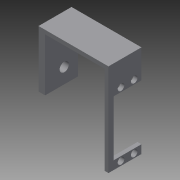
# Autodesk Inventor part: new_shoulder_2_modif
Saved by Autodesk Inventor 2014 SP1 (Build 180222100, 222)
## iProperties
Created: 2014-12-06
Part Number: new_shoulder_2_modif
Material: Générique
Document SubType Name: Modeling
Designer: astralien3000
Density: 1 g/cm^3
Appearance: Par défaut
d0: 45,000 mm
d1: 5,000 mm
d2: 3,000 mm
d3: 3,000 mm
d4: 40,000 mm
d5: 20,000 mm
d6: 22,500 mm
d7: 70,000 mm
d8: 25,000 mm
d9: 0,00 deg
d10: 21,000 mm
d11: 6,400 mm
d12: 6,400 mm
d13: 42,000 mm
d14: 5,000 mm
d15: 5,000 mm
d16: 5,000 mm
d17: 3,200 mm
d18: 3,200 mm
d19: 5,000 mm
d22: 6,400 mm
d23: 21,000 mm
d24: 42,000 mm
d25: 7,000 mm
d27: 10,000 mm
d29: 0,00 deg
d31: 0,00 deg
Author: astralien3000
Autodesk Inventor part; units mm, degrees
ref_plane "YZ Plane" through (0, 0, 0) normal (1, 0, 0) x (0, 1, 0)
ref_plane "XZ Plane" through (0, 0, 0) normal (0, 1, 0) x (-1, 0, 0)
ref_plane "XY Plane" through (0, 0, 0) normal (0, 0, 1) x (1, 0, 0)
sketch "Esquisse1" plane through (0, 0, 0) normal (0, 1, 0) x (-1, 0, 0)
  line L0 (-25.5, 23) -> (-22.5, 23)
  line L1 (-22.5, 23) -> (-22.5, -47)
  line L2 (-22.5, -47) -> (-25.5, -47)
  line L3 (-25.5, -47) -> (-25.5, 23)
  line L4 (-22.5, 23) -> (27.5, 23)
  line L5 (27.5, 23) -> (27.5, 20)
  line L6 (27.5, 20) -> (-22.5, 20)
  line L7 (-22.5, 20) -> (-22.5, 23)
  line L8 (27.5, 20) -> (22.5, 20)
  line L9 (22.5, 20) -> (22.5, -20)
  line L10 (22.5, -20) -> (27.5, -20)
  line L11 (27.5, -20) -> (27.5, 20)
  point P0 (0, 0)
  dimension "d0" = 45
  dimension "d1" = 5
  dimension "d2" = 3
  dimension "d3" = 3
  dimension "d4" = 40
  dimension "d5" = 20
  dimension "d6" = 22.5
  dimension "d7" = 70
  constraints: 24 end point, 6 parallel, 3 horizontal, 3 perpendicular
  measures "d0" distance between parallel lines of L1 L9
  measures "d1" distance between parallel lines of L9 L11
  measures "d2" distance between parallel lines of L6 L4
  measures "d3" distance between parallel lines of L3 L1
  measures "d4" distance between parallel lines of L6 L10
  measures "d5" distance from line of point (0, 0) L6
  measures "d6" distance from line of point (0, 0) L9
  measures "d7" distance between parallel lines of L0 L2
extrude "Extrusion1" add sketch "Esquisse1" along normal blind 25
sketch "Esquisse2" plane through (25.5, 0, 23) normal (1, 0, 0) x (0, 0, -1)
  line L0 (70, 0) -> (70, 25) projected
  line L1 (0, 25) -> (70, 25) projected
  line L2 (70, 25) -> (63.6, 25)
  line L3 (63.6, 25) -> (63.6, 4)
  line L4 (63.6, 4) -> (70, 4)
  line L5 (70, 4) -> (70, 25)
  line L6 (63.6, 4) -> (21.6, 4)
  line L7 (21.6, 4) -> (21.6, 25)
  line L8 (21.6, 25) -> (63.6, 25)
  line L9 (63.6, 25) -> (63.6, 4)
  line L10 (21.6, 4) -> (15.2, 4)
  line L11 (15.2, 4) -> (15.2, 25)
  line L12 (15.2, 25) -> (21.6, 25)
  line L13 (21.6, 25) -> (21.6, 4)
  line L14 (15.2, 14.5) -> (70, 14.5) construction
  circle A0 centre (18.4, 19.5) radius 2.5
  circle A1 centre (66.8, 19.5) radius 2.5
  circle A2 centre (18.4, 9.5) radius 2.5
  circle A3 centre (66.8, 9.5) radius 2.5
  point P0 (23, 0)
  dimension "d10" = 21
  dimension "d11" = 6.4
  dimension "d12" = 6.4
  dimension "d13" = 42
  dimension "d14" = 5
  dimension "d15" = 5
  dimension "d16" = 5
  dimension "d17" = 3.2
  dimension "d18" = 3.2
  dimension "d19" = 5
  constraints: 26 end point, 6 parallel, 4 centre point, 3 horizontal, 3 perpendicular, 2 midpoint, 2 point on line, 2 symmetric about line, 2 other
  measures "d10" distance between parallel lines of L8 L6
  measures "d11" distance between parallel lines of L0 L3
  measures "d12" distance between parallel lines of L11 L7
  measures "d13" distance between parallel lines of L13 L3
  measures "d14" diameter of A0
  measures "d15" diameter of A1
  measures "d16" distance from line of L14 A0.centre
  measures "d17" distance from line of L11 A0.centre
  measures "d18" distance from line of L0 A1.centre
  measures "d19" distance from line of L14 A1.centre
sketch "Esquisse3" plane through (25.5, 0, 23) normal (1, 0, 0) x (0, 0, -1)
  line L0 (0, 25) -> (70, 25) projected
  line L1 (21.6, 4) -> (63.6, 4)
  line L2 (63.6, 4) -> (63.6, 25)
  line L3 (63.6, 25) -> (21.6, 25)
  line L4 (21.6, 25) -> (21.6, 4)
  line L5 (63.6, 4) -> (70, 4)
  line L6 (70, 4) -> (70, 25)
  line L7 (70, 25) -> (63.6, 25)
  line L8 (63.6, 25) -> (63.6, 4)
  line L9 (21.6, 14.5) -> (63.6, 14.5) construction
  circle A0 centre (31.6, 14.5) radius 3.5
  point P0 (23, 0)
  dimension "d22" = 6.4
  dimension "d23" = 21
  dimension "d24" = 42
  dimension "d25" = 7
  dimension "d27" = 10
  constraints: 18 end point, 4 parallel, 2 horizontal, 2 midpoint, 2 perpendicular, 2 point on line, 1 centre point
  measures "d22" distance between parallel lines of L6 L8
  measures "d23" distance between parallel lines of L0 L1
  measures "d24" distance between parallel lines of L2 L4
  measures "d25" diameter of A0
  measures "d27" distance from line of L4 A0.centre
extrude "Extrusion3" cut sketch "Esquisse3" against normal through all contours A0
extrude "Extrusion4" cut sketch "Esquisse2" against normal up to surface (3 mm away) contours L6 L7 L1 L3 | A0 | A1 | A2 | A3
equation "\"d5\" = 0.5 * d4"
equation "\"d6\" = 0.5 * d0"
equation "\"d12\" = d11"
equation "\"d15\" = d14"
equation "\"d18\" = d17"
equation "\"d19\" = d16"
